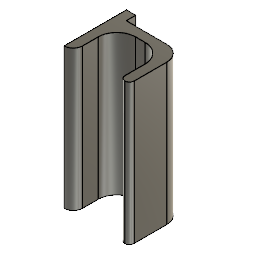
handle (Autodesk Fusion 360 design; units mm, degrees)
Autodesk Fusion 360 part; units mm, degrees
sketch "Sketch1" plane through (0, 0, 0) normal (0, 0, 1) x (1, 0, 0)
  line L0 (0, 20) -> (0, 0)
  line L1 (0, 0) -> (0, 0)
  line L2 (3, 3) -> (3, 7.9338)
  line L3 (9, 13.9338) -> (12, 13.9338)
  line L4 (18, 7.9338) -> (18, 1.5)
  line L5 (19.5, 0) -> (19.4638, 0)
  line L6 (20.9638, 1.5) -> (20.9638, 11.9338)
  line L7 (15.9638, 16.9338) -> (3, 16.9338)
  line L8 (3, 16.9338) -> (3, 20)
  line L9 (3, 20) -> (0, 20)
  arc A0 (20.9638, 11.9338) -> (15.9638, 16.9338) centre (15.9638, 11.9338) ccw
  arc A1 (18, 7.9338) -> (12, 13.9338) centre (12, 7.9338) ccw
  arc A2 (18, 1.5) -> (19.5, 0) centre (19.5, 1.5) ccw
  arc A3 (19.4638, 0) -> (20.9638, 1.5) centre (19.4638, 1.5) ccw
  arc A4 (9, 13.9338) -> (3, 7.9338) centre (9, 7.9338) ccw
  arc A5 (0, 0) -> (3, 3) centre (0, 3) ccw
  dimension "d1" = 5
  dimension "d2" = 6
  dimension "d3" = 1.5
  dimension "d4" = 1.5
  dimension "d5" = 3
  dimension "d6" = 3
  dimension "d7" = 2.9638
  dimension "d9" = 6
  dimension "d10" = 3
  dimension "d11" = 15
  dimension "d13" = 20
  measures "d1" radius of A0
  measures "d2" radius of A1
  measures "d3" radius of A2
  measures "d4" radius of A3
  measures "d5" distance of L0 L2
  measures "d6" distance of L3 L7
  measures "d7" distance of L4 L6
  measures "d9" radius of A4
  measures "d10" radius of A5
  measures "d11" distance of L2 L4
  measures "d13" distance of L0.end L9
extrude "Extrude1" add sketch "Sketch1" along normal blind 5
extrude "Extrude2" add 1 faces at (1.0204, 9.5959, 5) along direction (0, 0, 1) blind 40
